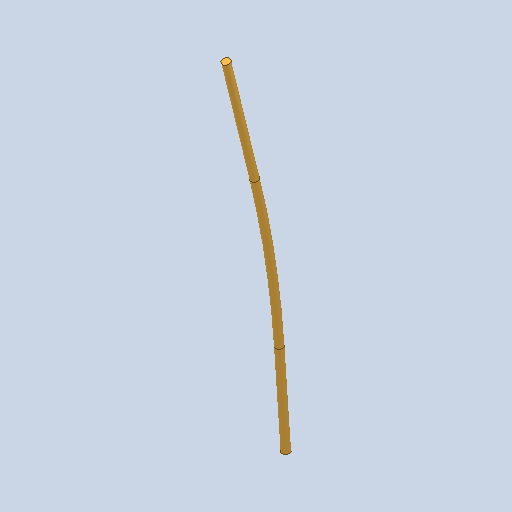
# Autodesk Inventor part: stuffing_tube
Saved by Autodesk Inventor 2022 (Build 260153070, 153G)
## iProperties
Created: 2021-05-28
Part Number: stuffing_tube
Material: Brass, Soft Yellow
Document SubType Name: Modeling
Designer: kardo
Density: 8.47 g/cm^3
Appearance: Brass - Satin
Author: kardo
Autodesk Inventor part; units mm, degrees
ref_plane "YZ Plane" through (0, 0, 0) normal (1, 0, 0) x (0, 1, 0)
ref_plane "XZ Plane" through (0, 0, 0) normal (0, 1, 0) x (-1, 0, 0)
ref_plane "XY Plane" through (0, 0, 0) normal (0, 0, 1) x (1, 0, 0)
derived "powertrain_outline.ipt"
sketch "sk_shaft_guide" plane through (6.24, 0, 0) normal (1, 0, 0) x (0, 1, 0)
  line L0 (-37.9005, 25.6108) -> (-277.6703, 19.7906) construction
  line L1 (-363, 18.496) -> (-297.6664, 19.4083) construction
  line L2 (94.8, 28.832) -> (28.4595, 27.2216) construction
  line L3 (28.4595, 27.2216) -> (-37.9005, 25.6108) construction
  line L4 (-485.3694, 0) -> (196.2166, 0) construction
  line L5 (-388, 0) -> (-328.1462, 4.1854)
  line L6 (-228.4098, 19.8341) -> (-155.2, 37.8624)
  arc A0 (-328.1462, 4.1854) -> (-228.4098, 19.8341) centre (-369.227, 591.669) ccw
  line L7 (-363, 18.496) -> (-388, 18.496) construction
  line L8 (-388, 18.496) -> (-388, 0) construction
  line L9 (-155.2, 37.8624) -> (-155.2, 16.279) construction
  line L10 (-158.5476, 51.4563) -> (-151.8524, 24.2685) construction
  line L11 (-151.8524, 24.2685) -> (-97.4769, 37.6588) construction
  line L12 (-97.4769, 37.6588) -> (-104.172, 64.8465) construction
  line L13 (-104.172, 64.8465) -> (-158.5476, 51.4563) construction
  line L14 (-158.5476, 51.4563) -> (-97.4769, 37.6588) construction
  line L15 (-151.8524, 24.2685) -> (-104.172, 64.8465) construction
  line L16 (-151.8524, 24.2685) -> (-151.8524, 19.2685) construction
  spline S0 degree 3 poles (-297.6664, 19.4083) (-291.0004, 19.5014) (-284.3349, 19.6288) (-277.6703, 19.7906) knots 0 0 0 0 1 1 1 1 construction
  spline S1 degree 4 poles (-297.6664, 19.4083) (-178.2238, 21.0761) (-46.6271, 18.3209) (53.0846, 11.363) (94.8, 28.832) knots 0 0 0 0 0 1 1 1 1 1 construction
  spline S2 degree 2 poles (0, 55.974) (-217.9618, 52.7695) (-363, 39.654) knots 0 0 0 1 1 1 construction
  spline S3 degree 4 poles (0, 55.974) (21.4177, 56.2889) (38.251, 53.3044) (69.464, 45.4203) (94.8, 37.536) knots 0 0 0 0 0 1 1 1 1 1 construction
  line L17 (-219.6703, 24.4386) -> (-238.3637, 19.8353) construction
  line L18 (-218.5316, 19.8143) -> (-237.2249, 15.211) construction
  line L19 (-238.3637, 19.8353) -> (-237.2249, 15.211) construction
  line L20 (-219.6703, 24.4386) -> (-218.5316, 19.8143) construction
  point P0 (0, 0)
  point P1 (-128.0122, 44.5575)
  point P2 (-128.0122, 44.5575)
  point P3 (-228.4098, 19.8341)
sketch "sk_shaft_profile" plane through (6.24, -155.2, 37.8624) normal (0, 0.9709921, 0.2391117) x (-1, 0, 0)
  circle A0 centre (0, 0) radius 2.3813
  point P0 (6.24, -73.8742)
sweep "Sweep1" add profiles "sk_shaft_profile" path "sk_shaft_guide" path curves L6 A0 L5
body "Solid1"
